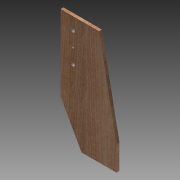
# Autodesk Inventor part: CNC-X-axis- side plates
Saved by Autodesk Inventor 2015 (Build 190159000, 159)
## iProperties
Created: 2015-03-24
Part Number: CNC-X-axis- side plates
Material: Generic
Document SubType Name: Modeling
Designer: Bangladesh
Density: 1 g/cm^3
Appearance: Default
Author: Bangladesh
Autodesk Inventor part; units mm, degrees
ref_plane "YZ Plane" through (0, 0, 0) normal (1, 0, 0) x (0, 1, 0)
ref_plane "XZ Plane" through (0, 0, 0) normal (0, 1, 0) x (-1, 0, 0)
ref_plane "XY Plane" through (0, 0, 0) normal (0, 0, 1) x (1, 0, 0)
sketch "Sketch1" plane through (0, 0, 0) normal (0, 0, 1) x (1, 0, 0)
  line L0 (-127.68, 259.036) -> (-127.68, -85.275)
  line L1 (-127.68, 259.036) -> (47.477, 259.036)
  line L2 (127.68, -259.036) -> (-32.32, -259.036)
  line L3 (-32.32, -259.036) -> (-127.68, -85.275)
  line L4 (127.68, -259.036) -> (127.68, -145.836)
  line L5 (127.68, -145.836) -> (47.477, 259.036)
  point P0 (0, 0)
  dimension "d6" = 344.311
  dimension "d7" = 175.157
  dimension "d9" = 160
  dimension "d10" = 113.2
  constraints: 12 end point, 1 horizontal
  measures "d6" distance of L0.start L0.end
  measures "d7" distance of L0.start L1.end
  measures "d9" distance of L2.start L2.end
  measures "d10" distance of L2.start L4.end
extrude "Extrusion1" add sketch "Sketch1" along normal mid plane 13
sketch "Sketch2" plane through (0, 0, 6.5) normal (0, 0, 1) x (1, 0, 0)
  circle A0 centre (-71.723, 203.108) radius 9
  circle A1 centre (-71.723, 69.5056) radius 9
  line L0 (47.477, 259.036) -> (-127.68, 259.036) projected
  line L1 (-127.68, 259.036) -> (-127.68, -85.275) projected
  circle A2 centre (-71.723, 136.306) radius 5
  point P0 (0, 0)
  dimension "d17" = 55.957
  dimension "d39" = 10
  dimension "d43" = 55.928
  dimension "d44" = 66.8004
  dimension "d45" = 66.802
  constraints: 3 centre point, 2 vertical alignment
  measures "d17" distance from line of L1 A1.centre
  measures "d39" diameter of A2
  measures "d43" distance from line of A0.centre L0
  measures "d44" distance of A1.centre A2.centre
  measures "d45" distance of A0.centre A2.centre
extrude "Extrusion4" cut sketch "Sketch2" against normal blind 25.4
body "Solid1"
